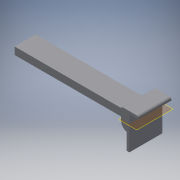
# Autodesk Inventor part: straightBar
Saved by Autodesk Inventor 2018 (Build 220112000, 112)
## iProperties
Created: 2017-12-09
Part Number: straightBar
Material: Generic
Document SubType Name: Modeling
Designer: kcmat
Density: 1 g/cm^3
Appearance: Default
Author: kcmat
Autodesk Inventor part; units mm, degrees
ref_plane "YZ Plane" through (0, 0, 0) normal (1, 0, 0) x (0, 1, 0)
ref_plane "XZ Plane" through (0, 0, 0) normal (0, 1, 0) x (-1, 0, 0)
ref_plane "XY Plane" through (0, 0, 0) normal (0, 0, 1) x (1, 0, 0)
sketch "Sketch1" plane through (0, 0, 0) normal (1, 0, 0) x (0, 1, 0)
  line L0 (0, 0) -> (7.62, 0)
  line L1 (7.62, 0) -> (7.62, -15.24)
  line L2 (7.62, -15.24) -> (0, -15.24)
  line L3 (0, -15.24) -> (0, 0)
  dimension "d0" = 7.62
  dimension "d1" = 15.24
  constraints: 8 end point, 2 parallel, 1 horizontal, 1 perpendicular
  measures "d0" distance of L1.end L2.end
  measures "d1" distance of L0.end L1.end
extrude "Extrusion1" add sketch "Sketch1" along normal blind 7.62
ref_plane "Work Plane1" through (0, 3.81, 0) normal (0, 1, 0) x (1, 0, 0)
sketch "Sketch3" plane through (0, 0, 0) normal (-1, 0, 0) x (0, 0, 1)
  line L0 (-2.7422, 2.1047) -> (-12.4487, 2.1047)
  line L1 (-12.4487, 2.1047) -> (-12.4487, 5.5015)
  line L2 (-12.4487, 5.5015) -> (-2.7422, 5.5015)
  line L3 (-2.7422, 5.5015) -> (-2.7422, 2.1047)
  point P0 (0, 0)
  constraints: 8 end point, 2 parallel, 1 horizontal, 1 perpendicular
extrude "Extrusion2" add sketch "Sketch3" along normal blind 1.27
sketch "Sketch4" plane through (0, 5.5015, -2.7422) normal (0, 1, 0) x (1, 0, 0)
  line L0 (-1.27, 9.7065) -> (-1.27, 0) projected
  line L1 (-1.27, 0) -> (-52.07, 0)
  line L2 (-52.07, 0) -> (-52.07, 9.7065)
  line L3 (-52.07, 9.7065) -> (-1.27, 9.7065)
  line L4 (-1.27, 9.7065) -> (-1.27, 0)
  point P0 (0, -2.7422)
  dimension "d6" = 50.8
  constraints: 8 end point, 2 parallel, 1 horizontal, 1 perpendicular
  measures "d6" distance of L2.end L3.end
extrude "Extrusion3" add sketch "Sketch4" against normal up to surface (3.3968 mm away)
sketch "Sketch5" plane through (7.62, 0, 0) normal (1, 0, 0) x (0, 0, -1)
  line L0 (15.24, 7.62) -> (15.24, 0) projected
  line L1 (0, 7.62) -> (15.24, 7.62) projected
  line L2 (15.24, 0) -> (0, 0)
  line L3 (0, 0) -> (0, 7.62)
  line L4 (0, 7.62) -> (15.24, 7.62)
  line L5 (15.24, 7.62) -> (15.24, 0)
  constraints: 8 end point, 2 parallel, 1 horizontal, 1 perpendicular
extrude "Extrusion4" cut sketch "Sketch5" against normal blind 3.81
sketch "Sketch6" plane through (0, 7.62, 0) normal (0, 1, 0) x (1, 0, 0)
  line L0 (0, 15.24) -> (3.81, 15.24) projected
  line L1 (0, 15.24) -> (8.0091, 15.24)
  line L2 (8.0091, 15.24) -> (8.0091, 0)
  line L3 (8.0091, 0) -> (0, 0)
  line L4 (0, 0) -> (0, 15.24)
  constraints: 8 end point, 2 parallel, 1 horizontal, 1 perpendicular
extrude "Extrusion5" add sketch "Sketch6" along normal blind 1.27
sketch "Sketch7" plane through (0, 0, 0) normal (0, 0, 1) x (1, 0, 0)
  line L0 (3.81, 0) -> (2.54, 0)
  line L1 (2.54, 0) -> (2.54, -7.62)
  line L2 (2.54, -7.62) -> (3.81, -7.62)
  line L3 (3.81, -7.62) -> (3.81, 0)
  point P0 (0, 0)
  dimension "d13" = 1.27
  dimension "d14" = 7.62
  constraints: 8 end point, 2 parallel, 1 horizontal, 1 perpendicular
  measures "d13" distance of L2.end L1.end
  measures "d14" distance of L1.end L0.end
extrude "Extrusion6" add sketch "Sketch7" against normal up to surface (15.24 mm away)
fillet "Fillet1" radius 3.175 5 edges at (0, 0, -7.62) (0, 3.8031, -2.7422) (0, 2.1047, -7.5954) (0, 3.8031, -12.4487) (0, 5.5015, -7.5954)
fillet "Fillet2" radius 1 1 edges at (8.0091, 8.89, -7.62)
fillet "Fillet3" radius 1 1 edges at (0, 8.89, -7.62)
body "Solid1"
